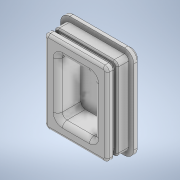
# Autodesk Inventor part: TAPA
Saved by Autodesk Inventor 2021 (Build 250183000, 183)
## iProperties
Created: 2022-05-04
Part Number: TAPA
Material: Genérico
Document SubType Name: Modeling
Designer: PC
Density: 1 g/cm^3
Appearance: Valor por defecto
Author: PC
Autodesk Inventor part; units mm, degrees
ref_plane "YZ Plane" through (0, 0, 0) normal (1, 0, 0) x (0, 1, 0)
ref_plane "XZ Plane" through (0, 0, 0) normal (0, 1, 0) x (-1, 0, 0)
ref_plane "XY Plane" through (0, 0, 0) normal (0, 0, 1) x (1, 0, 0)
sketch "Boceto1" plane through (0, 0, 0) normal (0, 0, 1) x (1, 0, 0)
  line L0 (-10.8323, 26.4321) -> (12.9177, 26.4321)
  line L1 (14.9177, 24.4321) -> (14.9177, -7.9479)
  line L2 (12.9177, -9.9479) -> (-10.8323, -9.9479)
  line L3 (-12.8323, -7.9479) -> (-12.8323, 24.4321)
  arc A0 (14.9177, 24.4321) -> (12.9177, 26.4321) centre (12.9177, 24.4321) ccw
  arc A1 (12.9177, -9.9479) -> (14.9177, -7.9479) centre (12.9177, -7.9479) ccw
  arc A2 (-12.8323, -7.9479) -> (-10.8323, -9.9479) centre (-10.8323, -7.9479) ccw
  arc A3 (-10.8323, 26.4321) -> (-12.8323, 24.4321) centre (-10.8323, 24.4321) ccw
  line L4 (12.9177, 28.4321) -> (-10.8323, 28.4321)
  arc A4 (-10.8323, 28.4321) -> (-14.8323, 24.4321) centre (-10.8323, 24.4321) ccw
  line L5 (-14.8323, 24.4321) -> (-14.8323, -7.9479)
  arc A5 (-14.8323, -7.9479) -> (-10.8323, -11.9479) centre (-10.8323, -7.9479) ccw
  line L6 (-10.8323, -11.9479) -> (12.9177, -11.9479)
  arc A6 (12.9177, -11.9479) -> (16.9177, -7.9479) centre (12.9177, -7.9479) ccw
  line L7 (16.9177, -7.9479) -> (16.9177, 24.4321)
  arc A7 (16.9177, 24.4321) -> (12.9177, 28.4321) centre (12.9177, 24.4321) ccw
  dimension "d17" = 27.75
  dimension "d18" = 36.38
  dimension "d19" = 2
  dimension "d20" = 2
  constraints: 16 end point, 16 point on circle, 8 centre point, 8 tangent, 4 parallel, 3 equal radius, 2 perpendicular, 1 horizontal, 7 other
  measures "d17" distance between parallel lines of L3 L1
  measures "d18" distance between parallel lines of L2 L0
  measures "d19" radius of A0
  measures "d20" distance between parallel lines of L0 L4
extrude "Extrusión5" add sketch "Boceto1" along normal blind 3
extrude "Extrusión6" add sketch "Boceto1" along normal blind 8 contours L0 A0 L1 A1 L2 A2 L3 A3
chamfer "Chaflán2" distance 1.5 angle 45 8 edges at (16.9177, 8.2421, 0) (15.7461, 27.2605, 0) (1.0427, 28.4321, 0) (-13.6607, 27.2605, 0) (-14.8323, 8.2421, 0) (-13.6607, -10.7763, 0) (1.0427, -11.9479, 0) (15.7461, -10.7763, 0)
sketch "Boceto4" plane through (0, 0, 8) normal (0, 0, 1) x (1, 0, 0)
  line L0 (9.9177, 21.4321) -> (-7.8323, 21.4321)
  line L1 (-7.8323, 21.4321) -> (-7.8323, -4.9479)
  line L2 (-7.8323, -4.9479) -> (9.9177, -4.9479)
  line L3 (9.9177, -4.9479) -> (9.9177, 21.4321)
  line L4 (14.9177, -7.9479) -> (14.9177, 24.4321) projected
  line L5 (-10.8323, -9.9479) -> (12.9177, -9.9479) projected
  line L6 (-12.8323, 24.4321) -> (-12.8323, -7.9479) projected
  line L7 (12.9177, 26.4321) -> (-10.8323, 26.4321) projected
  point P0 (0, 0)
  dimension "d31" = 5
  dimension "d32" = 5
  dimension "d33" = 5
  dimension "d34" = 5
  constraints: 8 end point, 2 parallel, 1 horizontal, 1 perpendicular
  measures "d31" distance between parallel lines of L3 L4
  measures "d32" distance between parallel lines of L5 L2
  measures "d33" distance between parallel lines of L6 L1
  measures "d34" distance between parallel lines of L7 L0
extrude "Extrusión7" cut sketch "Boceto4" against normal blind 5
sketch "Boceto5" plane through (0, 0, 8) normal (0, 0, 1) x (1, 0, 0)
  line L0 (-7.8323, -4.9479) -> (-7.8323, 21.4321) projected
  line L1 (9.9177, -4.9479) -> (-7.8323, -4.9479) projected
  line L2 (9.9177, 21.4321) -> (9.9177, -4.9479) projected
  line L3 (-7.8323, 21.4321) -> (9.9177, 21.4321) projected
  line L4 (11.5177, -8.5479) -> (-9.4323, -8.5479)
  line L5 (-11.4323, -6.5479) -> (-11.4323, 23.0321)
  line L6 (-9.4323, 25.0321) -> (11.5177, 25.0321)
  line L7 (13.5177, 23.0321) -> (13.5177, -6.5479)
  line L8 (14.9177, -7.9479) -> (14.9177, 24.4321) projected
  arc A0 (13.5177, 23.0321) -> (11.5177, 25.0321) centre (11.5177, 23.0321) ccw
  arc A1 (11.5177, -8.5479) -> (13.5177, -6.5479) centre (11.5177, -6.5479) ccw
  arc A2 (-11.4323, -6.5479) -> (-9.4323, -8.5479) centre (-9.4323, -6.5479) ccw
  arc A3 (-9.4323, 25.0321) -> (-11.4323, 23.0321) centre (-9.4323, 23.0321) ccw
  point P0 (0, 0)
  dimension "d37" = 1.4
  dimension "d38" = 2
  constraints: 8 end point, 8 point on circle, 8 tangent, 4 centre point, 3 equal radius, 3 other
  measures "d37" distance between parallel lines of L7 L8
  measures "d38" radius of A0
extrude "Extrusión8" add sketch "Boceto5" along normal blind 1.2
sketch "Boceto6" plane through (0, 0, 9.2) normal (0, 0, 1) x (1, 0, 0)
  arc A0 (13.5177, 23.0321) -> (11.5177, 25.0321) centre (11.5177, 23.0321) ccw projected
  line L0 (13.5177, 23.0321) -> (13.5177, -6.5479) projected
  arc A1 (11.5177, -8.5479) -> (13.5177, -6.5479) centre (11.5177, -6.5479) ccw projected
  line L1 (11.5177, -8.5479) -> (-9.4323, -8.5479) projected
  arc A2 (-11.4323, -6.5479) -> (-9.4323, -8.5479) centre (-9.4323, -6.5479) ccw projected
  line L2 (-11.4323, -6.5479) -> (-11.4323, 23.0321) projected
  arc A3 (-9.4323, 25.0321) -> (-11.4323, 23.0321) centre (-9.4323, 23.0321) ccw projected
  line L3 (-9.4323, 25.0321) -> (11.5177, 25.0321) projected
  line L4 (-10.8323, -9.9479) -> (12.9177, -9.9479) projected
  arc A4 (12.9177, -9.9479) -> (14.9177, -7.9479) centre (12.9177, -7.9479) ccw projected
  line L5 (14.9177, -7.9479) -> (14.9177, 24.4321) projected
  arc A5 (14.9177, 24.4321) -> (12.9177, 26.4321) centre (12.9177, 24.4321) ccw projected
  line L6 (12.9177, 26.4321) -> (-10.8323, 26.4321) projected
  arc A6 (-10.8323, 26.4321) -> (-12.8323, 24.4321) centre (-10.8323, 24.4321) ccw projected
  line L7 (-12.8323, 24.4321) -> (-12.8323, -7.9479) projected
  arc A7 (-12.8323, -7.9479) -> (-10.8323, -9.9479) centre (-10.8323, -7.9479) ccw projected
  point P0 (0, 0)
extrude "Extrusión9" add sketch "Boceto6" along normal blind 3 contours L0 A1 L1 A2 L2 A3 L3 A0 | A7 L7 A6 L6 A5 L5 A4 L4
chamfer "Chaflán3" distance 0.8 angle 45 8 edges at (14.3319, 25.8463, 9.2) (1.0427, 26.4321, 9.2) (-12.2465, 25.8463, 9.2) (-12.8323, 8.2421, 9.2) (-12.2465, -9.3621, 9.2) (1.0427, -9.9479, 9.2) (14.3319, -9.3621, 9.2) (14.9177, 8.2421, 9.2)
chamfer "Chaflán4" distance 0.8 angle 45 8 edges at (14.9177, 8.2421, 8) (14.3319, 25.8463, 8) (1.0427, 26.4321, 8) (-12.2465, 25.8463, 8) (-12.8323, 8.2421, 8) (-12.2465, -9.3621, 8) (1.0427, -9.9479, 8) (14.3319, -9.3621, 8)
sketch "Boceto8" plane through (0, 0, 12.2) normal (0, 0, 1) x (1, 0, 0)
  line L0 (-7.8323, 21.4321) -> (9.9177, 21.4321) projected
  line L1 (9.9177, 21.4321) -> (-6.7823, 21.4321)
  line L2 (-6.7823, 21.4321) -> (-6.7823, -4.6186)
  line L3 (-6.7823, -4.6186) -> (9.9177, -4.6186)
  line L4 (9.9177, -4.6186) -> (9.9177, 21.4321)
  point P0 (0, 0)
  point P1 (-6.7823, 21.4321)
  constraints: 8 end point, 2 parallel, 1 horizontal, 1 perpendicular
extrude "Extrusión11" add sketch "Boceto8" against normal blind 10
fillet "Empalme4" radius 1.5 8 edges at (-12.2465, 25.8463, 12.2) (-12.8323, 8.2421, 12.2) (-12.2465, -9.3621, 12.2) (1.0427, -9.9479, 12.2) (14.3319, -9.3621, 12.2) (14.9177, 8.2421, 12.2) (14.3319, 25.8463, 12.2) (1.0427, 26.4321, 12.2)
sketch "Boceto9" plane through (0, 0, 12.2) normal (0, 0, 1) x (1, 0, 0)
  arc A0 (-10.8323, 24.9321) -> (-11.3323, 24.4321) centre (-10.8323, 24.4321) ccw projected
  line L0 (-11.3323, -7.9479) -> (-11.3323, 24.4321) projected
  arc A1 (-11.3323, -7.9479) -> (-10.8323, -8.4479) centre (-10.8323, -7.9479) ccw projected
  line L1 (12.9177, -8.4479) -> (-10.8323, -8.4479) projected
  arc A2 (12.9177, -8.4479) -> (13.4177, -7.9479) centre (12.9177, -7.9479) ccw projected
  line L2 (13.4177, 24.4321) -> (13.4177, -7.9479) projected
  arc A3 (13.4177, 24.4321) -> (12.9177, 24.9321) centre (12.9177, 24.4321) ccw projected
  line L3 (-10.8323, 24.9321) -> (12.9177, 24.9321) projected
  line L4 (-6.8323, 20.4321) -> (8.9177, 20.4321)
  line L5 (8.9177, 20.4321) -> (8.9177, -3.9479)
  line L6 (8.9177, -3.9479) -> (-6.8323, -3.9479)
  line L7 (-6.8323, -3.9479) -> (-6.8323, 20.4321)
  point P0 (0, 0)
  dimension "d58" = 4.5
  constraints: 8 end point, 3 other
  measures "d58" distance between parallel lines of L7 L0
extrude "Extrusión12" cut sketch "Boceto9" against normal blind 10 contours L4 L5 L6 L7
sketch "Boceto10" plane through (0, 0, 0) normal (0, 0, -1) x (-1, 0, 0)
  line L0 (-3.4177, -6.7017) -> (-3.4177, 13.8603) construction
  line L1 (-3.4177, 13.8603) -> (2.7577, 13.8603) construction
  line L2 (2.7577, 13.8603) -> (2.7577, -6.7017) construction
  line L3 (2.7577, -6.7017) -> (-3.4177, -6.7017) construction
  line L4 (-15.4177, -7.9479) -> (-15.4177, 24.4321) projected
  line L5 (-3.4177, -6.0698) -> (-3.4177, -3.2835)
  spline S0 degree 2 poles (-3.4177, -3.2835) (-3.4177, -2.5819) (-3.2734, -1.7411) (-3.1142, -1.4923) knots 0 0 0 1 2 2 2
  spline S1 degree 2 poles (-3.1142, -1.4923) (-2.8505, -1.0793) (-1.9897, -0.6514) (-1.4325, -0.6514) knots 0 0 0 1 2 2 2
  spline S2 degree 2 poles (-1.4325, -0.6514) (-0.8852, -0.6514) (-0.099, -0.9997) (0.1597, -1.3579) knots 0 0 0 1 2 2 2
  spline S3 degree 2 poles (0.1597, -1.3579) (0.3687, -1.6565) (0.5478, -2.4327) (0.5478, -3.2337) knots 0 0 0 1 2 2 2
  line L6 (0.5478, -3.2337) -> (0.5478, -4.7861)
  line L7 (0.5478, -4.7861) -> (2.6823, -4.7861)
  line L8 (2.6823, -4.7861) -> (2.6823, -6.0698)
  line L9 (2.6823, -6.0698) -> (-3.4177, -6.0698)
  line L10 (-2.3281, -3.3034) -> (-2.3281, -4.7861)
  line L11 (-2.3281, -4.7861) -> (-0.5319, -4.7861)
  line L12 (-0.5319, -4.7861) -> (-0.5319, -3.2238)
  spline S4 degree 2 poles (-0.5319, -3.2238) (-0.5319, -2.6416) (-0.9747, -2.0794) (-1.4325, -2.0794) knots 0 0 0 1 2 2 2
  spline S5 degree 2 poles (-1.4325, -2.0794) (-1.9201, -2.0794) (-2.3281, -2.6317) (-2.3281, -3.3034) knots 0 0 0 1 2 2 2
  line L13 (-3.4177, 1.498) -> (0.2294, 1.498)
  spline S6 degree 2 poles (0.2294, 1.498) (1.0852, 1.498) (1.7618, 2.115) (1.7618, 2.8713) knots 0 0 0 1 2 2 2
  spline S7 degree 2 poles (1.7618, 2.8713) (1.7618, 3.6275) (1.0901, 4.2395) (0.2294, 4.2395) knots 0 0 0 1 2 2 2
  line L14 (0.2294, 4.2395) -> (-3.4177, 4.2395)
  line L15 (-3.4177, 4.2395) -> (-3.4177, 5.5232)
  line L16 (-3.4177, 5.5232) -> (0.2642, 5.5232)
  spline S8 degree 2 poles (0.2642, 5.5232) (0.911, 5.5232) (1.6822, 5.354) (1.9061, 5.165) knots 0 0 0 1 2 2 2
  spline S9 degree 2 poles (1.9061, 5.165) (2.339, 4.8018) (2.747, 3.6922) (2.747, 2.8713) knots 0 0 0 1 2 2 2
  spline S10 degree 2 poles (2.747, 2.8713) (2.747, 2.0503) (2.339, 0.9308) (1.9061, 0.5676) knots 0 0 0 1 2 2 2
  spline S11 degree 2 poles (1.9061, 0.5676) (1.6872, 0.3835) (0.9409, 0.2193) (0.2642, 0.2193) knots 0 0 0 1 2 2 2
  line L17 (0.2642, 0.2193) -> (-3.4177, 0.2193)
  line L18 (-3.4177, 0.2193) -> (-3.4177, 1.498)
  spline S12 degree 2 poles (2.6823, 9.1852) (2.6823, 8.3344) (2.3937, 7.5035) (2.0405, 7.1751) knots 0 0 0 1 2 2 2
  spline S13 degree 2 poles (2.0405, 7.1751) (1.727, 6.8716) (0.9309, 6.6228) (0.2095, 6.6228) knots 0 0 0 1 2 2 2
  line L19 (0.2095, 6.6228) -> (-3.4177, 6.6228)
  line L20 (-3.4177, 6.6228) -> (-3.4177, 7.9065)
  line L21 (-3.4177, 7.9065) -> (0.1647, 7.9065)
  spline S14 degree 2 poles (0.1647, 7.9065) (0.702, 7.9065) (1.1349, 8.001) (1.2693, 8.1155) knots 0 0 0 1 2 2 2
  spline S15 degree 2 poles (1.2693, 8.1155) (1.4832, 8.2996) (1.6673, 8.8319) (1.6673, 9.2996) knots 0 0 0 1 2 2 2
  line L22 (1.6673, 9.2996) -> (1.6673, 10.8072)
  line L23 (1.6673, 10.8072) -> (2.6823, 10.8072)
  line L24 (2.6823, 10.8072) -> (2.6823, 9.1852)
  line L25 (-2.3281, 16.6485) -> (-2.3281, 13.4791)
  spline S16 degree 2 poles (-2.3281, 13.4791) (-2.3281, 12.9666) (-1.9449, 12.489) (-1.532, 12.489) knots 0 0 0 1 2 2 2
  spline S17 degree 2 poles (-1.532, 12.489) (-1.2036, 12.489) (-0.8702, 12.897) (-0.8702, 13.3) knots 0 0 0 1 2 2 2
  line L26 (-0.8702, 13.3) -> (-0.8702, 14.9966)
  spline S18 degree 2 poles (-0.8702, 14.9966) (-0.8702, 16.0514) (-0.0741, 16.9421) (0.8563, 16.9421) knots 0 0 0 1 2 2 2
  spline S19 degree 2 poles (0.8563, 16.9421) (1.7967, 16.9421) (2.6823, 15.9121) (2.6823, 14.8125) knots 0 0 0 1 2 2 2
  line L27 (2.6823, 14.8125) -> (2.6823, 11.3943)
  line L28 (2.6823, 11.3943) -> (1.5927, 11.3943)
  line L29 (1.5927, 11.3943) -> (1.5927, 14.6085)
  spline S20 degree 2 poles (1.5927, 14.6085) (1.5927, 15.1558) (1.2742, 15.6036) (0.906, 15.6036) knots 0 0 0 1 2 2 2
  spline S21 degree 2 poles (0.906, 15.6036) (0.5229, 15.6036) (0.1995, 15.1907) (0.1995, 14.6931) knots 0 0 0 1 2 2 2
  line L30 (0.1995, 14.6931) -> (0.1995, 13.1806)
  spline S22 degree 2 poles (0.1995, 13.1806) (0.1995, 12.1257) (-0.6413, 11.1505) (-1.5519, 11.1505) knots 0 0 0 1 2 2 2
  spline S23 degree 2 poles (-1.5519, 11.1505) (-2.5221, 11.1505) (-3.4177, 12.1755) (-3.4177, 13.29) knots 0 0 0 1 2 2 2
  line L31 (-3.4177, 13.29) -> (-3.4177, 16.6485)
  line L32 (-3.4177, 16.6485) -> (-2.3281, 16.6485)
  spline S24 degree 2 poles (-2.3529, 20.4249) (-2.3529, 19.7284) (-1.6564, 19.0169) (-0.9399, 18.982) knots 0 0 0 1 2 2 2
  line L33 (-0.9399, 18.982) -> (-0.9349, 22.5296)
  line L34 (-0.9349, 22.5296) -> (0.1249, 22.5296)
  line L35 (0.1249, 22.5296) -> (0.1249, 18.9721)
  spline S25 degree 2 poles (0.1249, 18.9721) (0.921, 18.977) (1.6175, 19.6438) (1.6175, 20.4249) knots 0 0 0 1 2 2 2
  line L36 (1.6175, 20.4249) -> (1.6175, 22.5296)
  line L37 (1.6175, 22.5296) -> (2.6823, 22.5296)
  line L38 (2.6823, 22.5296) -> (2.6823, 20.3602)
  spline S26 degree 2 poles (2.6823, 20.3602) (2.6823, 19.6438) (2.4385, 18.8228) (2.1449, 18.4596) knots 0 0 0 1 2 2 2
  spline S27 degree 2 poles (2.1449, 18.4596) (1.7718, 17.9919) (0.5727, 17.5242) (-0.2582, 17.5242) knots 0 0 0 1 2 2 2
  spline S28 degree 2 poles (-0.2582, 17.5242) (-1.8803, 17.5242) (-3.4177, 18.9273) (-3.4177, 20.4001) knots 0 0 0 1 2 2 2
  line L39 (-3.4177, 20.4001) -> (-3.4177, 22.5296)
  line L40 (-3.4177, 22.5296) -> (-2.3529, 22.5296)
  line L41 (-2.3529, 22.5296) -> (-2.3529, 20.4249)
  point P0 (0, 0)
  dimension "d63" = 12
  constraints: 2 other
  measures "d63" distance between parallel lines of L0 L4
extrude "Extrusión13" cut sketch "Boceto10" against normal blind 0.35
sketch "Boceto11" plane through (0, 0, 12.2) normal (0, 0, 1) x (1, 0, 0)
  line L0 (14.9177, -7.9479) -> (14.9177, 24.4321) projected
  arc A0 (14.9177, 24.4321) -> (12.9177, 26.4321) centre (12.9177, 24.4321) ccw projected
  line L1 (12.9177, 26.4321) -> (-10.8323, 26.4321) projected
  arc A1 (-10.8323, 26.4321) -> (-12.8323, 24.4321) centre (-10.8323, 24.4321) ccw projected
  line L2 (-12.8323, 24.4321) -> (-12.8323, -7.9479) projected
  arc A2 (-12.8323, -7.9479) -> (-10.8323, -9.9479) centre (-10.8323, -7.9479) ccw projected
  line L3 (-10.8323, -9.9479) -> (12.9177, -9.9479) projected
  arc A3 (12.9177, -9.9479) -> (14.9177, -7.9479) centre (12.9177, -7.9479) ccw projected
  line L4 (-10.8323, 26.2521) -> (12.9177, 26.2521)
  arc A4 (14.7377, 24.4321) -> (12.9177, 26.2521) centre (12.9177, 24.4321) ccw
  line L5 (14.7377, 24.4321) -> (14.7377, -7.9479)
  arc A5 (12.9177, -9.7679) -> (14.7377, -7.9479) centre (12.9177, -7.9479) ccw
  line L6 (12.9177, -9.7679) -> (-10.8323, -9.7679)
  arc A6 (-12.6523, -7.9479) -> (-10.8323, -9.7679) centre (-10.8323, -7.9479) ccw
  line L7 (-12.6523, -7.9479) -> (-12.6523, 24.4321)
  arc A7 (-10.8323, 26.2521) -> (-12.6523, 24.4321) centre (-10.8323, 24.4321) ccw
  point P0 (0, 0)
  dimension "d66" = 0.18
  constraints: 8 end point, 8 point on circle, 4 centre point, 7 other
  measures "d66" distance between parallel lines of L1 L4
extrude "Extrusión14" cut sketch "Boceto11" against normal up to surface (9.2 mm away)
sketch "Boceto12" plane through (0, 0, 12.2) normal (0, 0, 1) x (1, 0, 0)
  line L0 (-6.8323, 20.048) -> (-8.3323, 20.048) projected
  line L1 (-8.3323, 20.048) -> (-8.3323, -3.5639) projected
  line L2 (-6.8323, -3.5639) -> (-8.3323, -3.5639) projected
  line L3 (-6.8323, -3.5639) -> (-6.8323, 20.048) projected
  line L4 (-6.7823, 20.4321) -> (-6.7823, 22.6743) projected
  arc A0 (-6.7823, 22.6743) -> (-8.3323, 20.048) centre (-5.3323, 20.048) ccw projected
  line L5 (-6.8323, 20.048) -> (-8.3323, 20.048) projected
  arc A1 (-6.7823, 20.4321) -> (-6.8323, 20.048) centre (-5.3323, 20.048) ccw projected
  line L6 (-6.8323, -3.5639) -> (-8.3323, -3.5639) projected
  arc A2 (-8.3323, -3.5639) -> (-6.7823, -6.1902) centre (-5.3323, -3.5639) ccw projected
  line L7 (-6.7823, -6.1902) -> (-6.7823, -3.9479) projected
  arc A3 (-6.8323, -3.5639) -> (-6.7823, -3.9479) centre (-5.3323, -3.5639) ccw projected
  point P0 (0, 0)
extrude "Extrusión15" add sketch "Boceto12" against normal up to surface (10 mm away)
sketch "Boceto13" plane through (0, 0, 12.2) normal (0, 0, 1) x (1, 0, 0)
  line L0 (8.9177, 20.4321) -> (8.9177, -3.9479) projected
  line L1 (-6.8323, -3.9479) -> (8.9177, -3.9479)
  line L2 (8.9177, -3.9479) -> (8.9177, 20.4321)
  line L3 (8.9177, 20.4321) -> (-6.8323, 20.4321)
  line L4 (-6.8323, 20.4321) -> (-6.8323, -3.9479)
  point P0 (0, 0)
  constraints: 8 end point, 2 parallel, 1 horizontal, 1 perpendicular
extrude "Extrusión16" cut sketch "Boceto13" against normal up to surface (10 mm away)
fillet "Empalme7" radius 2 4 edges at (-6.8323, 20.4321, 7.2) (-6.8323, -3.9479, 7.2) (8.9177, -3.9479, 7.2) (8.9177, 20.4321, 7.2)
fillet "Empalme8" radius 2 8 edges at (-6.2465, 19.8463, 12.2) (1.0427, 20.4321, 12.2) (8.3319, 19.8463, 12.2) (8.9177, 8.2421, 12.2) (8.3319, -3.3621, 12.2) (1.0427, -3.9479, 12.2) (-6.2465, -3.3621, 12.2) (-6.8323, 8.2421, 12.2)
